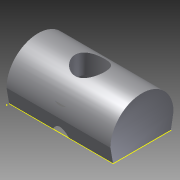
# Autodesk Inventor part: cam pivot
Saved by Autodesk Inventor 2012 (Build 160160000, 160)
## iProperties
Created: 2012-01-06
Part Number: cam pivot
Material: Default
Document SubType Name: Modeling
Designer: Kennell
Density: 1 g/cm^3
Author: Kennell
Autodesk Inventor part; units mm, degrees
ref_plane "YZ Plane" through (0, 0, 0) normal (1, 0, 0) x (0, 1, 0)
ref_plane "XZ Plane" through (0, 0, 0) normal (0, 1, 0) x (-1, 0, 0)
ref_plane "XY Plane" through (0, 0, 0) normal (0, 0, 1) x (1, 0, 0)
sketch "Sketch1" plane through (0, 0, 0) normal (0, 0, 1) x (1, 0, 0)
  line L0 (0, 0) -> (14, 0)
  line L1 (14, 0) -> (14, 8.5)
  line L2 (14, 8.5) -> (0, 8.5)
  line L3 (0, 8.5) -> (0, 0)
  dimension "d0" = 14
  dimension "d1" = 8.5
  constraints: 8 end point, 2 parallel, 1 horizontal, 1 perpendicular
  measures "d0" distance of L2.end L1.end
  measures "d1" distance of L1.end L0.end
extrude "Extrusion1" add sketch "Sketch1" along normal blind 2
sketch "Sketch2" plane through (14, 0, 0) normal (1, 0, 0) x (0, 0, -1)
  line L0 (-2, 8.5) -> (-2, 0) projected
  line L1 (0, 0) -> (-2, 0) projected
  line L2 (0, 8.5) -> (-2, 8.5) projected
  arc A0 (-2, 8.5) -> (-2, 0) centre (-2, 4.25) ccw
  line L3 (-2, 8.5) -> (-2, 0)
  constraints: 2 end point, 2 point on circle, 2 tangent, 1 centre point, 1 collinear
extrude "Extrusion2" add sketch "Sketch2" against normal blind 14
chamfer "Chamfer1" distance 2 angle 10 1 edges at (7, 0, 0) measured on face at (4.6667, 0, 0.6667)
chamfer "Chamfer2" distance 2 angle 10 1 edges at (7, 8.5, 0) measured on face at (9.3333, 8.5, 0.6667)
sketch "Sketch3" plane through (0, 0, 0) normal (0, 0, -1) x (-1, 0, 0)
  line L0 (-14, 8.1473) -> (0, 8.1473) projected
  line L1 (-14, 0.3527) -> (-14, 8.1473) projected
  line L2 (0, 0.3527) -> (-14, 0.3527) projected
  line L3 (0, 8.1473) -> (0, 0.3527) projected
  point P0 (0, 0)
hole "Hole1" at (7, 4.2527, 0) direction (0, 0, 1) diameter 4 end through all
hole "Hole2" at (7, 4.2527, 0) direction (0, 0, 1) diameter 8.1 depth 3.5
body "Solid1"
